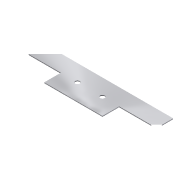
# Autodesk Inventor part: P_hips_001
Saved by Autodesk Inventor 2016 (Build 200138000, 138)
## iProperties
Created: 2016-02-23
Part Number: P_hips_001
Material: Aluminum 6061
Document SubType Name: Modeling
Designer: Mateusz
Density: 2.7 g/cm^3
Appearance: Aluminum - Flat
Author: Mateusz
Autodesk Inventor part; units mm, degrees
ref_plane "YZ Plane" through (0, 0, 0) normal (1, 0, 0) x (0, 1, 0)
ref_plane "XZ Plane" through (0, 0, 0) normal (0, 1, 0) x (-1, 0, 0)
ref_plane "XY Plane" through (0, 0, 0) normal (0, 0, 1) x (1, 0, 0)
derived "skeleton.ipt"
sketch "Sketch1" plane through (0, 0, 0) normal (0, 0, 1) x (1, 0, 0)
  line L0 (0, 56) -> (0, -56) projected
  line L1 (-224, 0) -> (224, 0) projected
  line L2 (150, 37.5) -> (-150, 37.5)
  line L3 (-150, 37.5) -> (-150, -37.5)
  line L4 (-150, -37.5) -> (150, -37.5)
  line L5 (150, -37.5) -> (150, 37.5)
  point P0 (0, 0)
  dimension "d1" = 300
  dimension "d2" = 75
  constraints: 8 end point, 2 parallel, 1 horizontal, 1 perpendicular, 2 other
  measures "d1" distance between parallel lines of L5 L3
  measures "d2" distance between parallel lines of L2 L4
extrude "Extrusion1" add sketch "Sketch1" along normal blind 2
sketch "Sketch2" plane through (0, 0, 0) normal (0, 0, -1) x (-1, 0, 0)
  line L0 (-150, 37.5) -> (150, 37.5) projected
  line L1 (-150, -37.5) -> (-150, 37.5) projected
  line L2 (150, -37.5) -> (-150, -37.5) projected
  line L3 (150, 37.5) -> (150, -37.5) projected
  line L4 (150, -37.5) -> (-150, -37.5) projected
  line L5 (0, -37.5) -> (0, 37.5)
  line L6 (150, 0) -> (-150, 0)
  line L7 (-150, -37.5) -> (-150, 37.5) projected
  point P0 (0, 0)
  point P1 (-30, 0)
  point P2 (30, 0)
  dimension "d5" = 60
  dimension "d13" = 0
  constraints: 4 end point, 4 midpoint, 1 symmetric about line
  measures "d5" distance of point (-30, 0) point (30, 0)
  measures "d13" distance from line of L6 point (-30, 0)
hole "Hole1" at (30, 0, 0) at (-30, 0, 0) direction (0, 0, 1) diameter 11 end through all
sketch "Sketch3" plane through (0, 0, 2) normal (0, 0, 1) x (1, 0, 0)
  line L0 (-212, 0) -> (222, 0) projected
  line L1 (0, 53) -> (0, -55.5) projected
  line L2 (150, -37.5) -> (75, -37.5)
  line L3 (75, -37.5) -> (75, 0)
  line L4 (75, 0) -> (150, 0)
  line L5 (150, 0) -> (150, -37.5)
  point P0 (0, 0)
  dimension "d14" = 75
  dimension "d15" = 150
  dimension "d16" = 37.5
  dimension "d18" = 0
  constraints: 8 end point, 2 parallel, 1 horizontal, 1 perpendicular
  measures "d14" distance between parallel lines of L1 L3
  measures "d15" distance between parallel lines of L1 L5
  measures "d16" distance between parallel lines of L0 L2
  measures "d18" distance between parallel lines of L0 L4
extrude "Extrusion2" cut sketch "Sketch3" against normal through all
mirror "Mirror1" about plane through (0, 0, 0) normal (1, 0, 0) of "Extrusion2"
equation "\"d1\" = hips_width"
equation "\"d2\" = hips_length"
equation "\"d5\" = leg_spc"
equation "\"d15\" = 0.5 * hips_width"
equation "\"d16\" = 0.5 * hips_length"
equation "\"hips_width\" = 300"
equation "\"hips_length\" = 75"
equation "\"leg_spc\" = 60"
body "Solid1"
